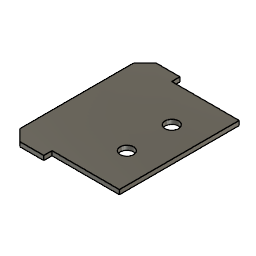
GPL H200 to H200G3 (Autodesk Fusion 360 design; units mm, degrees)
Autodesk Fusion 360 part; units mm, degrees
sketch "スケッチ1" plane through (0, 0, 0) normal (0, 0, 1) x (1, 0, 0)
  line L0 (-21.5, 91) -> (-68.5, 91)
  line L1 (-68.5, 91) -> (-68.5, -91)
  line L2 (-68.5, -91) -> (-21.5, -91)
  line L3 (68.5, -80) -> (68.5, 80)
  line L4 (60.2198, 80) -> (-68.5, -91) construction
  line L5 (-68.5, 91) -> (60.2198, -80) construction
  line L6 (-21.5, 91) -> (-21.5, 80)
  line L7 (-21.5, 80) -> (68.5, 80)
  line L8 (-21.5, -91) -> (-21.5, -80)
  line L9 (-21.5, -80) -> (68.5, -80)
  dimension "d2" = 182
  constraint horizontal L0
  constraint perpendicular L0 L1
  constraint parallel L0 L2
  constraint parallel L1 L3
  constraint coincident L4 origin
  constraint coincident L5 origin
  constraint vertical L6
  constraint horizontal L7
  constraint vertical L8
  constraint horizontal L9
  constraint coincident L7 L4.start
  constraint coincident L9 L5.end
  measures "d2" distance of L0.end L1.end
extrude "押し出し1" add sketch "スケッチ1" along normal blind 6
chamfer "面取り1" distance 15 angle 45 2 edges at (-68.5, -91, 3) (-68.5, 91, 3)
sketch "スケッチ2" plane through (0, 0, 6) normal (0, 0, 1) x (-1, 0, 0)
  line L0 (53.5, -91) -> (68.5, -76)
  line L1 (68.5, -76) -> (68.5, 76)
  line L2 (68.5, 76) -> (53.5, 91)
  line L3 (53.5, 91) -> (21.5, 91)
  line L4 (21.5, 91) -> (21.5, 80)
  line L5 (21.5, 80) -> (-68.5, 80)
  line L6 (-68.5, 80) -> (-68.5, -80)
  line L7 (-68.5, -80) -> (21.5, -80)
  line L8 (21.5, -80) -> (21.5, -91)
  line L9 (21.5, -91) -> (53.5, -91)
  line L10 (-68.5, -80) -> (-28.5, -80) construction
  line L11 (-28.5, -80) -> (-28.5, -30) construction
  line L12 (-28.5, -30) -> (-68.5, -30) construction
  line L13 (-68.5, -30) -> (-68.5, -80) construction
  line L14 (-68.5, 0) -> (91.4537, 0)
  point P0 (-28.5, -30)
  point P1 (-28.5, 30)
  dimension "d10" = 40
  dimension "d11" = 50
  constraint horizontal L10
  constraint vertical L11
  constraint horizontal L12
  constraint vertical L13
  constraint coincident L6.end L7.start
  constraint coincident P0 L11.end
  constraint midpoint L6 L14.start
  constraint perpendicular L6 L14
  constraint symmetric P0 L14 P1
  measures "d10" distance of L6.end L10.end
  measures "d11" distance of L6.end L12.end
hole "穴1" at (28.5, 30, 6) at (28.5, -30, 6) direction (0, 0, -1) diameter 18 end through all
